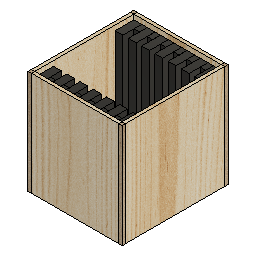
model (Autodesk Fusion 360 design; units mm, degrees)
Autodesk Fusion 360 part; units mm, degrees
note: some values were not read from the file. Chosen so that the rebuilt part matches the saved one: which bodies a step acts on.
sketch "Sketch1" plane through (0, 0, 0) normal (0, 0, 1) x (1, 0, 0) in component "box"
  line L0 (0, 0) -> (320.025, 0)
  line L1 (320.025, 0) -> (320.025, 363.15)
  line L2 (320.025, 363.15) -> (0, 363.15)
  line L3 (0, 363.15) -> (0, 0)
  line L4 (0, 363.15) -> (-12.7, 363.15)
  line L5 (-12.7, 363.15) -> (-12.7, 375.85)
  line L6 (-12.7, 375.85) -> (0, 375.85)
  line L7 (0, 375.85) -> (0, 363.15)
  line L8 (320.025, 363.15) -> (332.725, 363.15)
  line L9 (332.725, 363.15) -> (332.725, 375.85)
  line L10 (332.725, 375.85) -> (320.025, 375.85)
  line L11 (320.025, 375.85) -> (320.025, 363.15)
  line L12 (320.025, 0) -> (332.725, 0)
  line L13 (332.725, 0) -> (332.725, -12.7)
  line L14 (332.725, -12.7) -> (320.025, -12.7)
  line L15 (320.025, -12.7) -> (320.025, 0)
  line L16 (0, 0) -> (-12.7, 0)
  line L17 (-12.7, 0) -> (-12.7, -12.7)
  line L18 (-12.7, -12.7) -> (0, -12.7)
  line L19 (0, -12.7) -> (0, 0)
  line L20 (0, 363.15) -> (-12, 363.15)
  line L21 (-12, 363.15) -> (-12, 0)
  line L22 (-12, 0) -> (0, 0)
  line L23 (0, 0) -> (0, 363.15)
  line L24 (0, 0) -> (320.025, 0)
  line L25 (320.025, 0) -> (320.025, -12)
  line L26 (320.025, -12) -> (0, -12)
  line L27 (0, -12) -> (0, 0)
  line L28 (320.025, 0) -> (332.025, 0)
  line L29 (332.025, 0) -> (332.025, 363.15)
  line L30 (332.025, 363.15) -> (320.025, 363.15)
  line L31 (320.025, 363.15) -> (320.025, 0)
  line L32 (320.025, 363.15) -> (0, 363.15)
  line L33 (0, 363.15) -> (0, 375.15)
  line L34 (0, 375.15) -> (320.025, 375.15)
  line L35 (320.025, 375.15) -> (320.025, 363.15)
  line L36 (0, 363.15) -> (28.575, 363.15)
  line L37 (28.575, 363.15) -> (28.575, 294.575)
  line L38 (28.575, 294.575) -> (0, 294.575)
  line L39 (0, 294.575) -> (0, 363.15)
  line L40 (320.025, 363.15) -> (291.45, 363.15)
  line L41 (291.45, 363.15) -> (291.45, 294.575)
  line L42 (291.45, 294.575) -> (320.025, 294.575)
  line L43 (320.025, 294.575) -> (320.025, 363.15)
  line L44 (0, 0) -> (28.575, 0)
  line L45 (0, 54.2875) -> (0, 0)
  line L46 (320.025, 0) -> (291.45, 0)
  line L47 (320.025, 54.2875) -> (320.025, 0)
  line L48 (28.575, 363.15) -> (48.575, 363.15)
  line L49 (48.575, 363.15) -> (48.575, 334.575)
  line L50 (48.575, 334.575) -> (28.575, 334.575)
  line L51 (28.575, 334.575) -> (28.575, 363.15)
  line L52 (-12, 181.575) -> (332.025, 181.575) construction
  line L53 (48.575, 363.15) -> (77.15, 363.15)
  line L54 (77.15, 363.15) -> (77.15, 294.575)
  line L55 (77.15, 294.575) -> (48.575, 294.575)
  line L56 (48.575, 294.575) -> (48.575, 363.15)
  line L57 (77.15, 363.15) -> (97.15, 363.15)
  line L58 (97.15, 363.15) -> (97.15, 334.575)
  line L59 (97.15, 334.575) -> (77.15, 334.575)
  line L60 (77.15, 334.575) -> (77.15, 363.15)
  line L61 (97.15, 363.15) -> (125.725, 363.15)
  line L62 (125.725, 363.15) -> (125.725, 294.575)
  line L63 (125.725, 294.575) -> (97.15, 294.575)
  line L64 (97.15, 294.575) -> (97.15, 363.15)
  line L65 (125.725, 363.15) -> (145.725, 363.15)
  line L66 (145.725, 363.15) -> (145.725, 334.575)
  line L67 (145.725, 334.575) -> (125.725, 334.575)
  line L68 (125.725, 334.575) -> (125.725, 363.15)
  line L69 (145.725, 363.15) -> (174.3, 363.15)
  line L70 (174.3, 363.15) -> (174.3, 294.575)
  line L71 (174.3, 294.575) -> (145.725, 294.575)
  line L72 (145.725, 294.575) -> (145.725, 363.15)
  line L73 (174.3, 363.15) -> (194.3, 363.15)
  line L74 (194.3, 363.15) -> (194.3, 334.575)
  line L75 (194.3, 334.575) -> (174.3, 334.575)
  line L76 (174.3, 334.575) -> (174.3, 363.15)
  line L77 (194.3, 363.15) -> (222.875, 363.15)
  line L78 (222.875, 363.15) -> (222.875, 294.575)
  line L79 (222.875, 294.575) -> (194.3, 294.575)
  line L80 (194.3, 294.575) -> (194.3, 363.15)
  line L81 (222.875, 363.15) -> (242.875, 363.15)
  line L82 (242.875, 363.15) -> (242.875, 334.575)
  line L83 (242.875, 334.575) -> (222.875, 334.575)
  line L84 (222.875, 334.575) -> (222.875, 363.15)
  line L85 (242.875, 363.15) -> (271.45, 363.15)
  line L86 (271.45, 363.15) -> (271.45, 294.575)
  line L87 (271.45, 294.575) -> (242.875, 294.575)
  line L88 (242.875, 294.575) -> (242.875, 363.15)
  line L89 (271.45, 363.15) -> (291.45, 363.15)
  line L90 (291.45, 363.15) -> (291.45, 334.575)
  line L91 (291.45, 334.575) -> (271.45, 334.575)
  line L92 (271.45, 334.575) -> (271.45, 363.15)
  line L93 (0, 0) -> (28.575, 0)
  line L94 (28.575, 0) -> (28.575, 68.575)
  line L95 (28.575, 68.575) -> (0, 68.575)
  line L96 (0, 68.575) -> (0, 0)
  line L97 (28.575, 0) -> (48.575, 0)
  line L98 (48.575, 0) -> (48.575, 28.575)
  line L99 (48.575, 28.575) -> (28.575, 28.575)
  line L100 (28.575, 28.575) -> (28.575, 0)
  line L101 (48.575, 0) -> (77.15, 0)
  line L102 (77.15, 0) -> (77.15, 68.575)
  line L103 (77.15, 68.575) -> (48.575, 68.575)
  line L104 (48.575, 68.575) -> (48.575, 0)
  line L105 (77.15, 0) -> (97.15, 0)
  line L106 (97.15, 0) -> (97.15, 28.575)
  line L107 (97.15, 28.575) -> (77.15, 28.575)
  line L108 (77.15, 28.575) -> (77.15, 0)
  line L109 (97.15, 0) -> (125.725, 0)
  line L110 (125.725, 0) -> (125.725, 68.575)
  line L111 (125.725, 68.575) -> (97.15, 68.575)
  line L112 (97.15, 68.575) -> (97.15, 0)
  line L113 (125.725, 0) -> (145.725, 0)
  line L114 (145.725, 0) -> (145.725, 28.575)
  line L115 (145.725, 28.575) -> (125.725, 28.575)
  line L116 (125.725, 28.575) -> (125.725, 0)
  line L117 (145.725, 0) -> (174.3, 0)
  line L118 (174.3, 0) -> (174.3, 68.575)
  line L119 (174.3, 68.575) -> (145.725, 68.575)
  line L120 (145.725, 68.575) -> (145.725, 0)
  line L121 (174.3, 0) -> (194.3, 0)
  line L122 (194.3, 0) -> (194.3, 28.575)
  line L123 (194.3, 28.575) -> (174.3, 28.575)
  line L124 (174.3, 28.575) -> (174.3, 0)
  line L125 (194.3, 0) -> (222.875, 0)
  line L126 (222.875, 0) -> (222.875, 68.575)
  line L127 (222.875, 68.575) -> (194.3, 68.575)
  line L128 (194.3, 68.575) -> (194.3, 0)
  line L129 (222.875, 0) -> (242.875, 0)
  line L130 (242.875, 0) -> (242.875, 28.575)
  line L131 (242.875, 28.575) -> (222.875, 28.575)
  line L132 (222.875, 28.575) -> (222.875, 0)
  line L133 (242.875, 0) -> (271.45, 0)
  line L134 (271.45, 0) -> (271.45, 68.575)
  line L135 (271.45, 68.575) -> (242.875, 68.575)
  line L136 (242.875, 68.575) -> (242.875, 0)
  line L137 (271.45, 0) -> (291.45, 0)
  line L138 (291.45, 0) -> (291.45, 28.575)
  line L139 (291.45, 28.575) -> (271.45, 28.575)
  line L140 (271.45, 28.575) -> (271.45, 0)
  line L141 (291.45, 0) -> (320.025, 0)
  line L142 (320.025, 0) -> (320.025, 68.575)
  line L143 (320.025, 68.575) -> (291.45, 68.575)
  line L144 (291.45, 68.575) -> (291.45, 0)
  line L145 (28.575, 28.575) -> (48.575, 28.575)
  line L146 (48.575, 28.575) -> (48.575, 334.575)
  line L147 (48.575, 334.575) -> (28.575, 334.575)
  line L148 (28.575, 334.575) -> (28.575, 28.575)
  line L149 (77.15, 334.575) -> (97.15, 334.575)
  line L150 (97.15, 334.575) -> (97.15, 28.575)
  line L151 (97.15, 28.575) -> (77.15, 28.575)
  line L152 (77.15, 28.575) -> (77.15, 334.575)
  line L153 (125.725, 334.575) -> (145.725, 334.575)
  line L154 (145.725, 334.575) -> (145.725, 28.575)
  line L155 (145.725, 28.575) -> (125.725, 28.575)
  line L156 (125.725, 28.575) -> (125.725, 334.575)
  line L157 (174.3, 334.575) -> (194.3, 334.575)
  line L158 (194.3, 334.575) -> (194.3, 28.575)
  line L159 (194.3, 28.575) -> (174.3, 28.575)
  line L160 (174.3, 28.575) -> (174.3, 334.575)
  line L161 (222.875, 334.575) -> (242.875, 334.575)
  line L162 (242.875, 334.575) -> (242.875, 28.575)
  line L163 (242.875, 28.575) -> (222.875, 28.575)
  line L164 (222.875, 28.575) -> (222.875, 334.575)
  line L165 (271.45, 334.575) -> (291.45, 334.575)
  line L166 (291.45, 334.575) -> (291.45, 28.575)
  line L167 (291.45, 28.575) -> (271.45, 28.575)
  line L168 (271.45, 28.575) -> (271.45, 334.575)
  dimension "d9" = 363.15
  dimension "d15" = 320.025
  dimension "d16" = 12.7
  dimension "d17" = 12.7
  dimension "d18" = 12.7
  dimension "d19" = 12.7
  dimension "d20" = 12.7
  dimension "d21" = 12.7
  dimension "d22" = 12.7
  dimension "d23" = 12.7
  dimension "d24" = 12
  dimension "d25" = 12
  dimension "d26" = 12
  dimension "d27" = 12
  dimension "d29" = 28.575
  dimension "d30" = 68.575
  dimension "d31" = 68.575
  dimension "d32" = 28.575
  dimension "d37" = 20
  dimension "d38" = 28.575
  dimension "d41" = 28.575
  dimension "d42" = 68.575
  dimension "d43" = 28.575
  dimension "d44" = 28.575
  dimension "d45" = 28.575
  dimension "d46" = 28.575
  dimension "d47" = 20
  dimension "d48" = 20
  dimension "d49" = 20
  dimension "d50" = 20
  dimension "d51" = 28.575
  dimension "d52" = 28.575
  dimension "d53" = 28.575
  dimension "d54" = 28.575
  dimension "d55" = 28.575
  dimension "d56" = 68.575
  dimension "d57" = 68.575
  dimension "d58" = 68.575
  dimension "d59" = 68.575
  dimension "d60" = 68.575
  dimension "d61" = 68.575
  dimension "d62" = 68.575
  dimension "d63" = 68.575
  dimension "d64" = 68.575
  dimension "d65" = 68.575
  dimension "d66" = 68.575
  dimension "d67" = 28.575
  dimension "d68" = 28.575
  dimension "d69" = 28.575
  dimension "d70" = 28.575
  dimension "d71" = 28.575
  dimension "d72" = 28.575
  dimension "d73" = 28.575
  dimension "d74" = 28.575
  dimension "d75" = 20
  dimension "d76" = 20
  dimension "d77" = 20
  dimension "d78" = 20
  dimension "d79" = 20
  dimension "d80" = 20
  dimension "d81" = 28.575
  dimension "d82" = 28.575
  dimension "d83" = 28.575
  dimension "d84" = 28.575
  dimension "d85" = 28.575
  dimension "d86" = 20
  constraint horizontal L0
  constraint vertical L1
  constraint horizontal L2
  constraint vertical L3
  constraint coincident L0.start L3.end
  constraint horizontal L4
  constraint vertical L5
  constraint horizontal L6
  constraint vertical L7
  constraint horizontal L8
  constraint vertical L9
  constraint horizontal L10
  constraint vertical L11
  constraint horizontal L12
  constraint vertical L13
  constraint horizontal L14
  constraint vertical L15
  constraint horizontal L16
  constraint vertical L17
  constraint horizontal L18
  constraint vertical L19
  constraint horizontal L20
  constraint vertical L21
  constraint horizontal L22
  constraint vertical L23
  constraint coincident L16 L21.end
  constraint horizontal L24
  constraint vertical L25
  constraint horizontal L26
  constraint vertical L27
  constraint coincident L15 L25.end
  constraint horizontal L28
  constraint vertical L29
  constraint horizontal L30
  constraint vertical L31
  constraint coincident L8 L29.end
  constraint horizontal L32
  constraint vertical L33
  constraint horizontal L34
  constraint vertical L35
  constraint coincident L7 L33.end
  constraint horizontal L36
  constraint vertical L37
  constraint horizontal L38
  constraint vertical L39
  constraint horizontal L40
  constraint vertical L41
  constraint horizontal L42
  constraint vertical L43
  constraint horizontal L44
  constraint vertical L45
  constraint horizontal L46
  constraint vertical L47
  constraint horizontal L48
  constraint vertical L49
  constraint horizontal L50
  constraint vertical L51
  constraint midpoint L21 L52.start
  constraint midpoint L29 L52.end
  constraint horizontal L53
  constraint vertical L54
  constraint horizontal L55
  constraint vertical L56
  constraint horizontal L57
  constraint vertical L58
  constraint horizontal L59
  constraint vertical L60
  constraint horizontal L61
  constraint vertical L62
  constraint horizontal L63
  constraint vertical L64
  constraint horizontal L65
  constraint vertical L66
  constraint horizontal L67
  constraint vertical L68
  constraint horizontal L69
  constraint vertical L70
  constraint horizontal L71
  constraint vertical L72
  constraint horizontal L73
  constraint vertical L74
  constraint horizontal L75
  constraint vertical L76
  constraint horizontal L77
  constraint vertical L78
  constraint horizontal L79
  constraint vertical L80
  constraint horizontal L81
  constraint vertical L82
  constraint horizontal L83
  constraint vertical L84
  constraint horizontal L85
  constraint vertical L86
  constraint horizontal L87
  constraint vertical L88
  constraint horizontal L89
  constraint vertical L90
  constraint horizontal L91
  constraint vertical L92
  constraint coincident L41 L90.end
  constraint horizontal L93
  constraint vertical L94
  constraint horizontal L95
  constraint vertical L96
  constraint horizontal L97
  constraint vertical L98
  constraint horizontal L99
  constraint vertical L100
  constraint horizontal L101
  constraint vertical L102
  constraint horizontal L103
  constraint vertical L104
  constraint horizontal L105
  constraint vertical L106
  constraint horizontal L107
  constraint vertical L108
  constraint horizontal L109
  constraint vertical L110
  constraint horizontal L111
  constraint vertical L112
  constraint horizontal L113
  constraint vertical L114
  constraint horizontal L115
  constraint vertical L116
  constraint horizontal L117
  constraint vertical L118
  constraint horizontal L119
  constraint vertical L120
  constraint horizontal L121
  constraint vertical L122
  constraint horizontal L123
  constraint vertical L124
  constraint horizontal L125
  constraint vertical L126
  constraint horizontal L127
  constraint vertical L128
  constraint horizontal L129
  constraint vertical L130
  constraint horizontal L131
  constraint vertical L132
  constraint horizontal L133
  constraint vertical L134
  constraint horizontal L135
  constraint vertical L136
  constraint horizontal L137
  constraint vertical L138
  constraint horizontal L139
  constraint vertical L140
  constraint horizontal L141
  constraint vertical L142
  constraint horizontal L143
  constraint vertical L144
  constraint coincident L1 L142.end
  constraint horizontal L145
  constraint vertical L146
  constraint horizontal L147
  constraint vertical L148
  constraint horizontal L149
  constraint vertical L150
  constraint horizontal L151
  constraint vertical L152
  constraint horizontal L153
  constraint vertical L154
  constraint horizontal L155
  constraint vertical L156
  constraint horizontal L157
  constraint vertical L158
  constraint horizontal L159
  constraint vertical L160
  constraint horizontal L161
  constraint vertical L162
  constraint horizontal L163
  constraint vertical L164
  constraint horizontal L165
  constraint vertical L166
  constraint horizontal L167
  constraint vertical L168
  measures "d9" distance of L0.start L2.end
  measures "d15" distance of L1 L3
  measures "d16" distance of L2.end L4.end
  measures "d17" distance of L2.end L6.end
  measures "d18" distance of L1.end L8.end
  measures "d19" distance of L1.end L10.end
  measures "d20" distance of L0.end L14.end
  measures "d21" distance of L13 L15
  measures "d22" distance of L17 L19
  measures "d23" distance of L16 L18
  measures "d24" distance of L32 L34
  measures "d25" distance of L1 L29
  measures "d26" distance of L21 L23
  measures "d27" distance of L24 L26
  measures "d29" distance of L2.end L36.end
  measures "d30" distance of L2.end L38.end
  measures "d31" distance of L1.end L42.end
  measures "d32" distance of L1 L41
  measures "d37" distance of L36.end L48.end
  measures "d38" distance of L36.end L50.end
  measures "d41" distance of L48.end L53.end
  measures "d42" distance of L48.end L55.end
  measures "d43" distance of L62 L64
  measures "d44" distance of L70 L72
  measures "d45" distance of L78 L80
  measures "d46" distance of L86 L88
  measures "d47" distance of L54 L64
  measures "d48" distance of L62 L72
  measures "d49" distance of L70 L80
  measures "d50" distance of L78 L88
  measures "d51" distance of L32 L59
  measures "d52" distance of L2 L67
  measures "d53" distance of L2 L75
  measures "d54" distance of L32 L83
  measures "d55" distance of L2 L91
  measures "d56" distance of L32 L63
  measures "d57" distance of L32 L71
  measures "d58" distance of L2 L79
  measures "d59" distance of L2 L87
  measures "d60" distance of L0 L95
  measures "d61" distance of L0 L103
  measures "d62" distance of L24 L111
  measures "d63" distance of L0 L119
  measures "d64" distance of L0 L127
  measures "d65" distance of L24 L135
  measures "d66" distance of L0 L143
  measures "d67" distance of L24 L99
  measures "d68" distance of L24 L107
  measures "d69" distance of L24 L115
  measures "d70" distance of L24 L123
  measures "d71" distance of L24 L131
  measures "d72" distance of L0 L139
  measures "d73" distance of L31 L144
  measures "d74" distance of L3 L94
  measures "d75" distance of L134 L144
  measures "d76" distance of L126 L136
  measures "d77" distance of L118 L128
  measures "d78" distance of L110 L120
  measures "d79" distance of L102 L112
  measures "d80" distance of L94 L104
  measures "d81" distance of L102 L104
  measures "d82" distance of L134 L136
  measures "d83" distance of L126 L128
  measures "d84" distance of L118 L120
  measures "d85" distance of L150 L156
  measures "d86" distance of L41 L92
extrude "Extrude1" add sketch "Sketch1" along normal blind 381 contours L16 L17 L18 L19 L22 L27 | L4 L5 L6 L7 L20 L33 | L12 L13 L14 L15 L25 L28 | L8 L9 L10 L11 L30 L35 makes body 1 at (0, -8.4667, 127) makes body 2 at (-12.7, 367.3833, 127) makes body 3 at (328.4917, -12.7, 127) makes body 4 at (328.4917, 375.85, 127) in component "box"
extrude "Extrude2" add sketch "Sketch1" along normal blind 381 separate body contours L3 L4 L16 L20 L21 L22 L23 L39 L45 L96 | L0 L15 L19 L24 L25 L26 L27 L44 L46 L93 L97 L101 L105 L109 L113 L117 L121 L125 L129 L133 L137 L141 | L2 L7 L11 L32 L33 L34 L35 L36 L40 L48 L53 L57 L61 L65 L69 L73 L77 L81 L85 L89 | L1 L8 L12 L28 L29 L30 L31 L43 L47 L142 makes body 5 at (106.675, 0, 254) in component "box"
extrude "Extrude3" add sketch "Sketch1" along normal blind 362.9 and the other way blind -12 separate body contours L0 L3 L23 L24 L44 L45 L93 L94 L95 L96 L100 L148 | L0 L24 L98 L101 L102 L103 L104 L108 L146 L152 | L2 L3 L23 L32 L36 L37 L38 L39 L51 L148 | L0 L1 L24 L31 L46 L47 L138 L141 L142 L143 L144 L166 | L0 L24 L106 L109 L110 L111 L112 L116 L150 L156 | L2 L32 L49 L53 L54 L55 L56 L60 L146 L152 | L0 L24 L130 L133 L134 L135 L136 L140 L162 L168 | L0 L24 L114 L117 L118 L119 L120 L124 L154 L160 | L1 L2 L31 L32 L40 L41 L42 L43 L90 L166 | L2 L32 L58 L61 L62 L63 L64 L68 L150 L156 | L0 L24 L122 L125 L126 L127 L128 L132 L158 L164 | L2 L32 L82 L85 L86 L87 L88 L92 L162 L168 | L2 L32 L66 L69 L70 L71 L72 L76 L154 L160 | L2 L32 L74 L77 L78 L79 L80 L84 L158 L164 makes body 6 at (125.725, 340.2917, 128.9667) makes body 7 at (320.025, 317.4333, 128.9667) makes body 8 at (145.725, 22.8583, 245.9333) makes body 9 at (0, 45.7167, 245.9333) makes body 10 at (194.3, 22.8583, 245.9333) makes body 11 at (271.45, 340.2917, 128.9667) makes body 12 at (48.575, 317.4333, 245.9333) makes body 13 at (174.3, 340.2917, 128.9667) makes body 14 at (291.45, 22.8583, 245.9333) makes body 15 at (97.15, 22.8583, 245.9333) makes body 16 at (48.575, 22.8583, 245.9333) makes body 17 at (242.875, 22.8583, 245.9333) makes body 18 at (222.875, 340.2917, 128.9667) makes body 19 at (0, 340.2917, 128.9667) in component "box"
extrude "Extrude4" add sketch "Sketch1" along normal blind 363 and the other way blind -12 separate body contours L0 L24 L94 L97 L98 L99 L100 L104 L145 | L0 L24 L102 L105 L106 L107 L108 L112 L151 | L2 L32 L37 L48 L49 L50 L51 L56 L147 | L0 L24 L134 L137 L138 L139 L140 L144 L167 | L0 L24 L110 L113 L114 L115 L116 L120 L155 | L2 L32 L54 L57 L58 L59 L60 L64 L149 | L0 L24 L126 L129 L130 L131 L132 L136 L163 | L0 L24 L118 L121 L122 L123 L124 L128 L159 | L2 L32 L41 L86 L89 L90 L91 L92 L165 | L2 L32 L62 L65 L66 L67 L68 L72 L153 | L2 L32 L78 L81 L82 L83 L84 L88 L161 | L2 L32 L70 L73 L74 L75 L76 L80 L157 makes body 20 at (174.3, 353.625, 129) makes body 21 at (28.575, 9.525, 129) makes body 22 at (222.875, 9.525, 129) makes body 23 at (174.3, 9.525, 129) makes body 24 at (48.575, 353.625, 129) makes body 25 at (222.875, 353.625, 129) makes body 26 at (125.725, 353.625, 129) makes body 27 at (77.15, 9.525, 129) makes body 28 at (271.45, 9.525, 129) makes body 29 at (125.725, 9.525, 129) makes body 30 at (97.15, 353.625, 129) makes body 31 at (271.45, 353.625, 129) in component "box"
extrude "Extrude5" add sketch "Sketch1" along normal blind 40.575 and the other way blind -12 separate body contours L37 L50 L56 L94 L99 L104 L145 L146 L147 L148 | L54 L59 L64 L102 L107 L112 L149 L150 L151 L152 | L41 L86 L91 L134 L139 L144 L165 L166 L167 L168 | L62 L67 L72 L110 L115 L120 L153 L154 L155 L156 | L78 L83 L88 L126 L131 L136 L161 L162 L163 L164 | L70 L75 L80 L118 L123 L128 L157 L158 L159 L160 makes body 32 at (174.3, 130.575, 21.525) makes body 33 at (28.575, 130.575, 21.525) makes body 34 at (222.875, 130.575, 21.525) makes body 35 at (125.725, 130.575, 21.525) makes body 36 at (77.15, 130.575, 21.525) makes body 37 at (291.45, 232.575, 21.525) in component "box"
extrude "Extrude6" add sketch "Sketch1" along normal blind 12 separate body contours L0 L3 L23 L24 L44 L45 L93 L94 L95 L96 L100 L148 | L0 L24 L94 L97 L98 L99 L100 L104 L145 | L0 L24 L98 L101 L102 L103 L104 L108 L146 L152 | L37 L50 L56 L94 L99 L104 L145 L146 L147 L148 | L3 L23 L38 L95 L148 | L0 L24 L102 L105 L106 L107 L108 L112 L151 | L2 L3 L23 L32 L36 L37 L38 L39 L51 L148 | L0 L1 L24 L31 L46 L47 L138 L141 L142 L143 L144 L166 | L0 L24 L106 L109 L110 L111 L112 L116 L150 L156 | L54 L59 L64 L102 L107 L112 L149 L150 L151 L152 | L55 L103 L146 L152 | L2 L32 L37 L48 L49 L50 L51 L56 L147 | L0 L24 L134 L137 L138 L139 L140 L144 L167 | L0 L24 L110 L113 L114 L115 L116 L120 L155 | L2 L32 L49 L53 L54 L55 L56 L60 L146 L152 | L0 L24 L130 L133 L134 L135 L136 L140 L162 L168 | L41 L86 L91 L134 L139 L144 L165 L166 L167 L168 | L1 L31 L42 L143 L166 | L0 L24 L114 L117 L118 L119 L120 L124 L154 L160 | L62 L67 L72 L110 L115 L120 L153 L154 L155 L156 | L63 L111 L150 L156 | L2 L32 L54 L57 L58 L59 L60 L64 L149 | L1 L2 L31 L32 L40 L41 L42 L43 L90 L166 | L0 L24 L126 L129 L130 L131 L132 L136 L163 | L0 L24 L118 L121 L122 L123 L124 L128 L159 | L2 L32 L58 L61 L62 L63 L64 L68 L150 L156 | L2 L32 L41 L86 L89 L90 L91 L92 L165 | L0 L24 L122 L125 L126 L127 L128 L132 L158 L164 | L78 L83 L88 L126 L131 L136 L161 L162 L163 L164 | L87 L135 L162 L168 | L70 L75 L80 L118 L123 L128 L157 L158 L159 L160 | L71 L119 L154 L160 | L2 L32 L62 L65 L66 L67 L68 L72 L153 | L2 L32 L82 L85 L86 L87 L88 L92 L162 L168 | L2 L32 L66 L69 L70 L71 L72 L76 L154 L160 | L2 L32 L78 L81 L82 L83 L84 L88 L161 | L79 L127 L158 L164 | L2 L32 L70 L73 L74 L75 L76 L80 L157 | L2 L32 L74 L77 L78 L79 L80 L84 L158 L164 makes body 38 in component "box"
sketch "Sketch1 (2)" plane through (0, 0, 381) normal (0, 0, 1) x (-1, 0, 0) in component "lid"
  line L0 (-332.025, 0) -> (-332.025, -363.15)
  line L1 (-332.025, -363.15) -> (-320.025, -363.15)
  line L2 (-320.025, -363.15) -> (-320.025, 0)
  line L3 (-320.025, 0) -> (-332.025, 0)
  line L4 (0, 0) -> (-320.025, 0)
  line L5 (-320.025, 0) -> (-320.025, -363.15)
  line L6 (-320.025, -363.15) -> (0, -363.15)
  line L7 (0, -363.15) -> (0, 0)
  line L8 (12.7, 12.7) -> (-332.725, 12.7)
  line L9 (-332.725, 12.7) -> (-332.725, -375.85)
  line L10 (-332.725, -375.85) -> (12.7, -375.85)
  line L11 (12.7, -375.85) -> (12.7, 12.7)
  line L12 (-317.025, -3) -> (-317.025, -360.15)
  line L13 (-317.025, -360.15) -> (-3, -360.15)
  line L14 (-3, -360.15) -> (-3, -3)
  line L15 (-3, -3) -> (-317.025, -3)
  line L16 (-317.025, -360.15) -> (-267.025, -360.15)
  line L17 (-267.025, -360.15) -> (-267.025, -310.15)
  line L18 (-267.025, -310.15) -> (-317.025, -310.15)
  line L19 (-317.025, -310.15) -> (-317.025, -360.15)
  line L20 (-3, -360.15) -> (-53, -360.15)
  line L21 (-53, -360.15) -> (-53, -310.15)
  line L22 (-53, -310.15) -> (-3, -310.15)
  line L23 (-3, -310.15) -> (-3, -360.15)
  line L24 (-317.025, -3) -> (-267.025, -3)
  line L25 (-267.025, -3) -> (-267.025, -53)
  line L26 (-267.025, -53) -> (-317.025, -53)
  line L27 (-317.025, -53) -> (-317.025, -3)
  line L28 (-3, -3) -> (-53, -3)
  line L29 (-53, -3) -> (-53, -53)
  line L30 (-53, -53) -> (-3, -53)
  line L31 (-3, -53) -> (-3, -3)
  dimension "d106" = 12.7
  dimension "d107" = 12.7
  dimension "d108" = 12.7
  dimension "d109" = 12.7
  dimension "d111" = -3
  dimension "d153" = 50
  dimension "d154" = 50
  dimension "d155" = 50
  dimension "d156" = 50
  dimension "d157" = 50
  dimension "d158" = 50
  dimension "d159" = 50
  dimension "d160" = 50
  constraint horizontal L4
  constraint vertical L5
  constraint horizontal L6
  constraint vertical L7
  constraint coincident L1.end L2.start
  constraint coincident L4.start L7.end
  constraint horizontal L8
  constraint vertical L9
  constraint horizontal L10
  constraint vertical L11
  constraint horizontal L16
  constraint vertical L17
  constraint horizontal L18
  constraint vertical L19
  constraint horizontal L20
  constraint vertical L21
  constraint horizontal L22
  constraint vertical L23
  constraint horizontal L24
  constraint vertical L25
  constraint horizontal L26
  constraint vertical L27
  constraint horizontal L28
  constraint vertical L29
  constraint horizontal L30
  constraint vertical L31
  measures "d106" distance of L5 L9
  measures "d107" distance of L6 L10
  measures "d108" distance of L4 L8
  measures "d109" distance of L7 L11
  measures "d153" distance of L12.end L18.end
  measures "d154" distance of L13.end L20.end
  measures "d155" distance of L13.end L22.end
  measures "d156" distance of L12.start L24.end
  measures "d157" distance of L12.start L26.end
  measures "d158" distance of L14.end L30.end
  measures "d159" distance of L14 L29
  measures "d160" distance of L17 L19
extrude "Extrude1'" add sketch "Sketch1 (2)" against normal blind 18 separate body contours L12 L15 L24 L25 L26 L27 | L12 L13 L16 L17 L18 L19 | L14 L15 L28 L29 L30 L31 | L13 L14 L20 L21 L22 L23 makes body 39 at (300.3583, 343.4833, 381) makes body 40 at (300.3583, 19.6667, 381) makes body 41 at (19.6667, 343.4833, 381) makes body 42 at (19.6667, 36.3333, 381) in component "lid"
extrude "Extrude7" add sketch "Sketch1 (2)" along normal blind 18 separate body contours L0 L1 L2 L3 L5 | L2 L4 L5 L6 L7 | L8 L9 L10 L11 | L12 L15 L24 L25 L26 L27 | L12 L13 L14 L15 L17 L18 L21 L22 L25 L26 L29 L30 | L12 L13 L16 L17 L18 L19 | L14 L15 L28 L29 L30 L31 | L13 L14 L20 L21 L22 L23 makes body 43 in component "box"
copy_body "CutPasteBodies1" bodies 43 removing the originals makes body 44 in component "lid"
sketch "Sketch2" plane through (0, -12.7, 0) normal (0, -1, 0) x (1, 0, 0)
  line L0 (320.025, 0) -> (332.725, 0)
  line L1 (332.725, 0) -> (332.725, 381)
  line L2 (332.725, 381) -> (320.025, 381)
  line L3 (320.025, 381) -> (320.025, 0)
  circle A0 centre (326.025, 367) radius 3
  circle A1 centre (326.025, 343) radius 3
  circle A2 centre (326.025, 283) radius 3
  circle A3 centre (326.025, 26) radius 3
  circle A4 centre (326.025, 98) radius 3
  line L4 (326.025, 381) -> (326.025, 0) construction
  circle A5 centre (326.025, 211) radius 3
  circle A6 centre (326.025, 170) radius 3
  line L5 (160.0125, 381) -> (160.0125, 0) construction
  line L6 (0, 381) -> (320.025, 381) construction
  line L7 (320.025, 0) -> (0, 0) construction
  circle A7 centre (-6, 26) radius 3
  circle A8 centre (-6, 98) radius 3
  circle A9 centre (-6, 211) radius 3
  circle A10 centre (-6, 343) radius 3
  circle A11 centre (-6, 367) radius 3
  circle A12 centre (-6, 283) radius 3
  circle A13 centre (-6, 170) radius 3
  dimension "d116" = 6
  dimension "d120" = 14
  dimension "d122" = 6
  dimension "d123" = 24
  dimension "d125" = 6
  dimension "d127" = 60
  dimension "d132" = 6
  dimension "d133" = 6
  dimension "d134" = 26
  dimension "d135" = 72
  dimension "d136" = 6
  dimension "d137" = 6
  dimension "d138" = 6
  dimension "d139" = 72
  dimension "d140" = 72
  constraint coincident L2 L4.start
  constraint coincident L0 L4.end
  constraint perpendicular L0 L4
  constraint coincident A3.centre L4
  constraint coincident A4.centre L4
  constraint coincident A2.centre L4
  constraint coincident A1.centre L4
  constraint coincident A0.centre L4
  constraint coincident L4 A5.centre
  constraint coincident L4 A6.centre
  constraint parallel L3 L5
  constraint midpoint L5.start L6
  constraint midpoint L5.end L7
  constraint symmetric A0 L5 A11
  constraint symmetric A1 L5 A10
  constraint symmetric A2 L5 A12
  constraint symmetric A3 L5 A7
  constraint symmetric A4 L5 A8
  constraint symmetric A5 L5 A9
  constraint symmetric A6 L5 A13
  measures "d116" diameter of A0
  measures "d120" distance of L2 A0.centre
  measures "d122" diameter of A1
  measures "d123" vertical distance of A0.centre A1.centre
  measures "d125" diameter of A2
  measures "d127" vertical distance of A1.centre A2.centre
  measures "d132" diameter of A3
  measures "d133" diameter of A4
  measures "d134" distance of L0 A3.centre
  measures "d135" vertical distance of A3.centre A4.centre
  measures "d136" distance of L3 L4
  measures "d137" diameter of A5
  measures "d138" diameter of A6
  measures "d139" distance of A4.centre A6.centre
  measures "d140" distance of A2.centre A5.centre
sketch "Sketch3" plane through (0, -12, 0) normal (0, -1, 0) x (1, 0, 0)
  line L0 (0, 0) -> (320.025, 0)
  line L1 (320.025, 0) -> (320.025, 381)
  line L2 (320.025, 381) -> (0, 381)
  line L3 (0, 381) -> (0, 0)
  line L4 (0, 6) -> (320.025, 6) construction
  circle A0 centre (14, 6) radius 3
  circle A1 centre (306.025, 6) radius 3
  circle A2 centre (86, 6) radius 3
  circle A3 centre (234.025, 6) radius 3
  line L5 (320.025, 381) -> (320.025, 0) construction
  circle A4 centre (158, 6) radius 3
  dimension "d141" = 6
  dimension "d142" = 6
  dimension "d143" = 6
  dimension "d144" = 6
  dimension "d145" = 6
  dimension "d146" = 72
  dimension "d147" = 72
  dimension "d148" = 14
  dimension "d149" = 14
  dimension "d150" = 6
  dimension "d151" = 72
  constraint coincident L3 L4.start
  constraint coincident L1 L4.end
  constraint perpendicular L1 L4
  constraint coincident L4 A0.centre
  constraint coincident L4 A1.centre
  constraint coincident L4 A2.centre
  constraint coincident L4 A3.centre
  constraint coincident L4 A4.centre
  measures "d141" distance of L0 L4
  measures "d142" diameter of A0
  measures "d143" diameter of A1
  measures "d144" diameter of A2
  measures "d145" diameter of A3
  measures "d146" distance of A0.centre A2.centre
  measures "d147" distance of A1.centre A3.centre
  measures "d148" distance of L4.start A0.centre
  measures "d149" distance of A1.centre L5
  measures "d150" diameter of A4
  measures "d151" distance of A2.centre A4.centre
copy_body "CutPasteBodies1'" bodies 5 removing the originals makes body 45 in component "faces"
copy_body "CutPasteBodies2" bodies 38 removing the originals makes body 46 in component "faces"
copy_body "CutPasteBodies1''" bodies 4 2 1 3 removing the originals makes body 47 makes body 48 makes body 49 makes body 50 in component "corners"
copy_body "CutPasteBodies1'''" bodies 37 21 26 28 29 17 13 14 15 18 20 30 31 32 33 34 35 16 19 10 7 11 8 23 24 25 22 36 12 9 6 27 removing the originals makes body 51 makes body 52 makes body 53 makes body 54 makes body 55 makes body 56 makes body 57 makes body 58 makes body 59 makes body 60 makes body 61 makes body 62 makes body 63 makes body 64 makes body 65 makes body 66 makes body 67 makes body 68 makes body 69 makes body 70 makes body 71 makes body 72 makes body 73 makes body 74 makes body 75 makes body 76 makes body 77 makes body 78 makes body 79 makes body 80 makes body 81 makes body 82 in component "foam"
chamfer "Chamfer1" distance 5 angle 45 16 edges at (53, 28, 363) (28, 53, 363) (28, 3, 363) (3, 28, 363) (53, 335.15, 363) (28, 360.15, 363) (28, 310.15, 363) (3, 335.15, 363) (292.025, 53, 363) (317.025, 28, 363) (292.025, 3, 363) (267.025, 28, 363) (317.025, 335.15, 363) (292.025, 360.15, 363) (292.025, 310.15, 363) (267.025, 335.15, 363) on bodies 39 40 41 42 in component "lid"
component "box" placed x (1, 0, 0) y (0, 1, 0) z (0, 0, 1) at (0, 0, 0)
component "lid" placed x (1, 0, 0) y (0, 1, 0) z (0, 0, 1) at (0, 0, 0)
component "foam" placed x (1, 0, 0) y (0, 1, 0) z (0, 0, 1) at (0, 0, 0) in component "box"
component "corners" placed x (1, 0, 0) y (0, 1, 0) z (0, 0, 1) at (0, 0, 0) in component "box"
component "faces" placed x (1, 0, 0) y (0, 1, 0) z (0, 0, 1) at (0, 0, 0) in component "box"
equation "numberOfLeafs = 6"
equation "leafWidth = 306 mm"
equation "leafHeight = 1105 mm"
equation "leafThickness = 20 mm"
equation "stockFoamThickness = 1 1/8\""
equation "plyThickness = 12 mm"
equation "squareDowelThickness = ( 0.5 ) * 1 in"
equation "d9 = leafWidth + 2 * sideFoamThickness"
equation "dowelDiameter = 6 mm"
equation "bottomFoamThickness = stockFoamThickness"
equation "frontFoamThickness = stockFoamThickness"
equation "betweenFoamThickness = stockFoamThickness"
equation "sideFoamThickness = stockFoamThickness"
equation "d15 = 2 * frontFoamThickness + numberOfLeafs * leafThickness + ( numberOfLeafs - 1 ) * betweenFoamThickness"
equation "d16 = squareDowelThickness"
equation "d17 = squareDowelThickness"
equation "d18 = squareDowelThickness"
equation "d19 = squareDowelThickness"
equation "d20 = squareDowelThickness"
equation "d21 = squareDowelThickness"
equation "d22 = squareDowelThickness"
equation "d23 = squareDowelThickness"
equation "d24 = plyThickness"
equation "d25 = plyThickness"
equation "d26 = plyThickness"
equation "d27 = plyThickness"
equation "foamOverlap = 40 mm + sideFoamThickness"
equation "d29 = frontFoamThickness"
equation "d30 = foamOverlap"
equation "d31 = foamOverlap"
equation "d32 = frontFoamThickness"
equation "d37 = leafThickness"
equation "d38 = sideFoamThickness"
equation "d41 = betweenFoamThickness"
equation "d42 = foamOverlap"
equation "d43 = betweenFoamThickness"
equation "d44 = betweenFoamThickness"
equation "d45 = betweenFoamThickness"
equation "d46 = betweenFoamThickness"
equation "d47 = leafThickness"
equation "d48 = leafThickness"
equation "d49 = leafThickness"
equation "d50 = leafThickness"
equation "d51 = sideFoamThickness"
equation "d52 = sideFoamThickness"
equation "d53 = sideFoamThickness"
equation "d54 = sideFoamThickness"
equation "d55 = sideFoamThickness"
equation "d56 = foamOverlap"
equation "d57 = foamOverlap"
equation "d58 = foamOverlap"
equation "d59 = foamOverlap"
equation "d60 = foamOverlap"
equation "d61 = foamOverlap"
equation "d62 = foamOverlap"
equation "d63 = foamOverlap"
equation "d64 = foamOverlap"
equation "d65 = foamOverlap"
equation "d66 = foamOverlap"
equation "d67 = sideFoamThickness"
equation "d68 = sideFoamThickness"
equation "d69 = sideFoamThickness"
equation "d70 = sideFoamThickness"
equation "d71 = sideFoamThickness"
equation "d72 = sideFoamThickness"
equation "d73 = frontFoamThickness"
equation "d74 = frontFoamThickness"
equation "d75 = leafThickness"
equation "d76 = leafThickness"
equation "d77 = leafThickness"
equation "d78 = leafThickness"
equation "d79 = leafThickness"
equation "d80 = leafThickness"
equation "d81 = betweenFoamThickness"
equation "d82 = betweenFoamThickness"
equation "d83 = betweenFoamThickness"
equation "d84 = betweenFoamThickness"
equation "boxHeight = 15 in"
equation "d88 = boxHeight"
equation "d90 = boxHeight"
equation "d92 = boxHeight - lidPlyThickness - smidge"
equation "d94 = -plyThickness"
equation "d96 = boxHeight - lidPlyThickness"
equation "d98 = -plyThickness"
equation "d100 = bottomFoamThickness + plyThickness"
equation "d102 = -plyThickness"
equation "d104 = plyThickness"
equation "d106 = squareDowelThickness"
equation "d107 = squareDowelThickness"
equation "d108 = squareDowelThickness"
equation "d109 = squareDowelThickness"
equation "totalLidTolerance = 6 mm"
equation "d111 = -totalLidTolerance / 2"
equation "d112 = -lidPlyThickness"
equation "d114 = lidPlyThickness"
equation "d116 = dowelDiameter"
equation "dowelSpacing = 12 mm"
equation "dowelSpacingEdge = 14 mm"
equation "dowelOffset = 6 mm"
equation "d120 = dowelSpacingEdge"
equation "d122 = dowelDiameter"
equation "d123 = dowelSpacing * 2"
equation "d125 = dowelDiameter"
equation "d127 = dowelSpacing * 5"
equation "smidge = 0.1 mm"
equation "d132 = dowelDiameter"
equation "d133 = dowelDiameter"
equation "d134 = dowelSpacingEdge + dowelSpacing"
equation "d135 = dowelSpacing * 6"
equation "d136 = dowelOffset"
equation "d137 = dowelDiameter"
equation "d138 = dowelDiameter"
equation "d139 = dowelSpacing * 6"
equation "d140 = dowelSpacing * 6"
equation "d141 = dowelOffset"
equation "d142 = dowelDiameter"
equation "d143 = dowelDiameter"
equation "d144 = dowelDiameter"
equation "d145 = dowelDiameter"
equation "d146 = dowelSpacing * 6"
equation "d147 = dowelSpacing * 6"
equation "d148 = dowelSpacingEdge"
equation "d149 = dowelSpacingEdge"
equation "d150 = dowelDiameter"
equation "d151 = dowelSpacing * 6"
equation "lidAlignSize = 50 mm"
equation "d159 = lidAlignSize"
equation "d160 = lidAlignSize"
equation "lidAlignChamfer = 5 mm"
equation "d162 = lidAlignChamfer"
equation "lidPlyThickness = 18 mm"
named bodies: "Body1 (1)"
